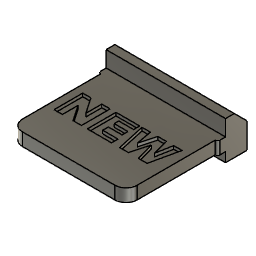
Nintendo 3DS - Cap v31 NEW (Autodesk Fusion 360 design; units mm, degrees)
Autodesk Fusion 360 part; units mm, degrees
note: some values were not read from the file. Set by a fixed rule: which sketch regions a step uses.
sketch "Boceto1" plane through (0, 0, 0) normal (0, 0, 1) x (1, 0, 0)
  line L0 (0, 0) -> (-3.6, 0)
  line L1 (-3.6, 0.6) -> (-3.6, 5.6)
  line L2 (-3.6, 5.6) -> (-3.75, 5.6)
  line L3 (0, 7.45) -> (-3.75, 7.45)
  line L4 (-3.75, 7.45) -> (-3.75, 5.6)
  line L5 (0, 1.75) -> (0, 22.5)
  line L6 (3.75, 7.45) -> (3.75, 5.6)
  line L7 (3.6, 5.6) -> (3.75, 5.6)
  line L8 (0, 0) -> (3.6, 0)
  line L9 (0, 7.45) -> (3.75, 7.45)
  line L10 (3.6, 0.6) -> (3.6, 5.6)
  line L11 (-3.75, 6.1) -> (0, 6.1)
  line L12 (3.75, 6.1) -> (0, 6.1)
  line L13 (-3.6, 0.6) -> (-3.6, 0)
  line L14 (3.6, 0.6) -> (3.6, 0)
  point P0 (3.6, 0.3)
  dimension "d1" = 3.6
  dimension "d2" = 5.6
  dimension "d4" = 3.75
  dimension "d8" = 6.1
  dimension "d25" = 1.35
  dimension "d26" = 0.5
  dimension "d28" = 0.3
  constraint coincident L0.start L8.start
  constraint horizontal L0
  constraint perpendicular L0 L1
  constraint perpendicular L1 L2
  constraint horizontal L3
  constraint perpendicular L2 L4
  constraint symmetric L0.start L5 L8.start
  constraint symmetric L0.end L5 L8.end
  constraint symmetric L1.end L5 L7.start
  constraint symmetric L3.start L5 L9.start
  constraint symmetric L3.end L5 L6.start
  constraint symmetric L2.end L5 L6.end
  constraint coincident L4 L11.start
  constraint coincident L5 L11.end
  constraint perpendicular L5 L11
  constraint symmetric L5 L11.start L12.start
  constraint symmetric L5 L11.end L12.end
  constraint coincident L10 P0
  constraint symmetric L5 L10.start L1.start
  constraint perpendicular L0 L13
  measures "d1" distance of L0.start L0.end
  measures "d2" distance of L0.end L1.end
  measures "d4" distance of L3.start L3.end
  measures "d8" vertical distance of L0.end L11.start
  measures "d25" distance of L3.end L11
  measures "d26" distance of L2.end L11.start
  measures "d28" distance of L8.end P0
extrude "Extruir2" add sketch "Boceto1" along normal blind 0.8 contours L0 L1 L2 L4 L6 L7 L8 L10 L11 L12 L13 L14
extrude "Extruir3" add sketch "Boceto1" along normal blind 1.8 contours L3 L4 L5 L11 | L5 L6 L9 L12
extrude "Extruir4" add sketch "Boceto1" against normal blind 0.6 contours L3 L4 L5 L11 | L5 L6 L9 L12
sketch "Boceto2" plane through (0, 0, 0) normal (0, 0, -1) x (1, 0, 0)
  line L0 (-3.75, -6.1) -> (3.75, -6.1)
  line L1 (3.75, -6.1) -> (3.75, -5.6)
  line L2 (3.75, -5.6) -> (3.6, -5.6)
  line L3 (3.6, -5.6) -> (3.6, -0.6)
  line L4 (3.6, 0) -> (-3.6, 0)
  line L5 (-3.6, -0.6) -> (-3.6, -5.6)
  line L6 (-3.6, -5.6) -> (-3.75, -5.6)
  line L7 (-3.75, -5.6) -> (-3.75, -6.1)
  line L8 (3, -1.6) -> (-3, -1.6) construction
  line L9 (-3, -1.6) -> (-3, -4.6) construction
  line L10 (-3, -4.6) -> (3, -4.6) construction
  line L11 (3, -4.6) -> (3, -1.6) construction
  arc A0 (3.6, -0.6) -> (3.6, 0) centre (3.6, -0.3) ccw
  arc A1 (-3.6, 0) -> (-3.6, -0.6) centre (-3.6, -0.3) ccw
  dimension "d15" = 1
  dimension "d21" = 1.5
  dimension "d22" = 3
  measures "d21" distance of L0.end
extrude "Extruir5" [suppressed]
sketch "Boceto3" plane through (0, 0, 0.8) normal (0, 0, 1) x (-1, 0, 0)
  line L0 (3.6, 0) -> (-3.6, 0)
  line L1 (-3.6, 0) -> (-3.6, -5.6)
  line L2 (-3.6, -5.6) -> (-3.75, -5.6)
  line L3 (-3.75, -5.6) -> (-3.75, -6.1)
  line L4 (-3.75, -6.1) -> (3.75, -6.1)
  line L5 (3.75, -6.1) -> (3.75, -5.6)
  line L6 (3.75, -5.6) -> (3.6, -5.6)
  line L7 (3.6, -5.6) -> (3.6, 0)
  line L8 (3, -1.6) -> (-3.0001, -1.6008) construction
  line L9 (-3.0001, -1.6008) -> (-2.9997, -4.6008) construction
  line L10 (-2.9997, -4.6008) -> (3.0004, -4.6) construction
  line L11 (3.0004, -4.6) -> (3, -1.6) construction
  dimension "d18" = 1.8
  dimension "d23" = 1.5
  dimension "d24" = 3
  text T0 "NEW" font "Arial Black" height 1.8 bold align centre middle in box 6.0001 x 3 at (3, -1.6) x (-1, -0.00013) y (0.00013, -1) spacing 1
  measures "d23" distance of L4.end
extrude "Extruir6" cut sketch "Boceto3" against normal blind 0.2 text T0
chamfer "Chaflán1" distance 0.8 angle 45 1 edges at (0, 7.45, 1.8)
fillet "Empalme1" radius 0.15 2 edges at (3.75, 5.6, 0.4) (-3.75, 5.6, 0.4)
fillet "Empalme2" radius 0.7 2 edges at (-3.6, 0, 0.4) (3.6, 0, 0.4)
equation "d11 = 0.8 mm + 1 mm"
